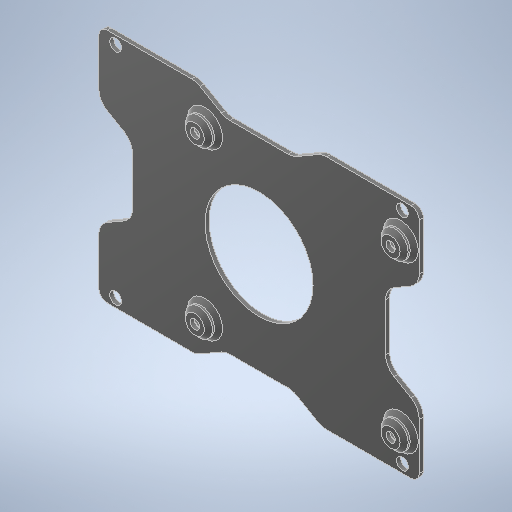
# Autodesk Inventor part: 3D_circuit-fix_raspberrypi
Saved by Autodesk Inventor 2025.1 (Build 291241020, 241B)
## iProperties
Created: 2024-07-24
Part Number: 3D_circuit-fix_raspberrypi
Material: 一般
Document SubType Name: Modeling
Designer: 8326d
Density: 1 g/cm^3
Appearance: 滑らか - 黒
Author: 8326d
## iProperties of the stored document 3D_circuit-fix_raspberrypi_3D プリント.ipt
Created: 2024-08-08
Part Number: 3D_circuit-fix_raspberrypi_3D プリント
Material: 一般
Document SubType Name: Modeling
Designer: 8326d
Density: 1 g/cm^3
Appearance: 既定
Author: 8326d
Autodesk Inventor part; units mm, degrees
ref_plane "YZ Plane" through (0, 0, 0) normal (1, 0, 0) x (0, 1, 0)
ref_plane "XZ Plane" through (0, 0, 0) normal (0, 1, 0) x (-1, 0, 0)
ref_plane "XY Plane" through (0, 0, 0) normal (0, 0, 1) x (1, 0, 0)
sketch "スケッチ1" plane through (0, 0, 0) normal (0, 0, 1) x (1, 0, 0)
  line L0 (-47.5, -35) -> (47.5, -35)
  line L1 (47.5, -35) -> (47.5, 35)
  line L2 (47.5, 35) -> (-47.5, 35)
  line L3 (-47.5, 35) -> (-47.5, -35)
  line L4 (-47.5, -35) -> (47.5, 35) construction
  line L5 (47.5, -35) -> (-47.5, 35) construction
  point P0 (0, 0)
  dimension "d0" = 95
  dimension "d1" = 70
  constraints: 12 end point, 2 midpoint, 2 parallel, 1 horizontal, 1 perpendicular
  measures "d0" distance of L2.end L1.end
  measures "d1" distance of L1.end L0.end
extrude "押し出し1" add sketch "スケッチ1" along normal blind 1.2
sketch "スケッチ2" plane through (0, 0, 1.2) normal (0, 0, 1) x (1, 0, 0)
  line L0 (-42.5, -32.5) -> (42.5, -32.5) construction
  line L1 (42.5, -32.5) -> (42.5, 32.5) construction
  line L2 (42.5, 32.5) -> (-42.5, 32.5) construction
  line L3 (-42.5, 32.5) -> (-42.5, -32.5) construction
  line L4 (-42.5, -32.5) -> (42.5, 32.5) construction
  line L5 (42.5, -32.5) -> (-42.5, 32.5) construction
  point P0 (0, 0)
  dimension "d4" = 85
  dimension "d5" = 65
  constraints: 12 end point, 2 midpoint, 2 parallel, 1 horizontal, 1 perpendicular
  measures "d4" distance of L2.end L1.end
  measures "d5" distance of L1.end L0.end
hole "穴1" at (-42.5, 32.5, 1.2) at (-42.5, -32.5, 1.2) at (42.5, -32.5, 1.2) at (42.5, 32.5, 1.2) direction (0, 0, -1) diameter 3.5 end through all
sketch "スケッチ3" plane through (0, 0, 1.2) normal (0, 0, 1) x (1, 0, 0)
  circle A0 centre (-16, -24.5) radius 4
  circle A1 centre (-16, 24.5) radius 4
  circle A2 centre (42, 24.5) radius 4
  circle A3 centre (42, -24.5) radius 4
  point P0 (0, 0)
  dimension "d13" = 8
  dimension "d14" = 8
  dimension "d15" = 8
  dimension "d16" = 8
  dimension "d17" = 49
  dimension "d21" = 58
  dimension "d22" = 24.5
  dimension "d52" = 16
  constraints: 4 centre point, 2 horizontal alignment, 2 vertical alignment
  measures "d13" diameter of A0
  measures "d14" diameter of A1
  measures "d15" diameter of A2
  measures "d16" diameter of A3
  measures "d17" distance of A0.centre A1.centre
  measures "d21" distance of A3.centre A0.centre
  measures "d22" vertical distance of A0.centre point (0, 0)
  measures "d52" horizontal distance of point (0, 0) A1.centre
extrude "押し出し2" add sketch "スケッチ3" along normal blind 3
chamfer "面取り1" distance 1.2 angle 45 8 edges at (-20, -24.5, 4.2) (-20, 24.5, 4.2) (38, 24.5, 4.2) (38, -24.5, 4.2) (-20, 24.5, 1.2) (-20, -24.5, 1.2) (38, 24.5, 1.2) (38, -24.5, 1.2)
sketch "スケッチ4" plane through (-16, -24.5, 4.2) normal (0, 0, 1) x (1, 0, 0)
  circle A0 centre (0, 49) radius 2.8 projected
  circle A1 centre (0, 0) radius 2.8 projected
  circle A2 centre (58, 0) radius 2.8 projected
  circle A3 centre (58, 49) radius 2.8 projected
  point P0 (16, 24.5)
hole "穴2" at (-16, 24.5, 4.2) at (-16, -24.5, 4.2) at (42, -24.5, 4.2) at (42, 24.5, 4.2) direction (0, 0, -1) diameter 2.8 end through all
sketch "スケッチ5" plane through (0, 0, 0) normal (0, 0, -1) x (-1, 0, 0)
  circle A0 centre (16, -24.5) radius 1.4 projected
  circle A1 centre (16, 24.5) radius 1.4 projected
  circle A2 centre (-42, 24.5) radius 1.4 projected
  circle A3 centre (-42, -24.5) radius 1.4 projected
  line L0 (16, -27.4445) -> (13.45, -25.9722)
  line L1 (13.45, -25.9722) -> (13.45, -23.0278)
  line L2 (13.45, -23.0278) -> (16, -21.5555)
  line L3 (16, -21.5555) -> (18.55, -23.0278)
  line L4 (18.55, -23.0278) -> (18.55, -25.9722)
  line L5 (18.55, -25.9722) -> (16, -27.4445)
  line L6 (16, 21.5555) -> (13.45, 23.0278)
  line L7 (13.45, 23.0278) -> (13.45, 25.9722)
  line L8 (13.45, 25.9722) -> (16, 27.4445)
  line L9 (16, 27.4445) -> (18.55, 25.9722)
  line L10 (18.55, 25.9722) -> (18.55, 23.0278)
  line L11 (18.55, 23.0278) -> (16, 21.5555)
  circle A4 centre (-42, -24.5) radius 2.8 projected
  line L12 (-42, -27.4445) -> (-44.55, -25.9722)
  line L13 (-44.55, -25.9722) -> (-44.55, -23.0278)
  line L14 (-44.55, -23.0278) -> (-42, -21.5555)
  line L15 (-42, -21.5555) -> (-39.45, -23.0278)
  line L16 (-39.45, -23.0278) -> (-39.45, -25.9722)
  line L17 (-39.45, -25.9722) -> (-42, -27.4445)
  line L18 (-42, 21.5555) -> (-44.55, 23.0278)
  line L19 (-44.55, 23.0278) -> (-44.55, 25.9722)
  line L20 (-44.55, 25.9722) -> (-42, 27.4445)
  line L21 (-42, 27.4445) -> (-39.45, 25.9722)
  line L22 (-39.45, 25.9722) -> (-39.45, 23.0278)
  line L23 (-39.45, 23.0278) -> (-42, 21.5555)
  point P0 (0, 0)
  dimension "d36" = 5.1
  dimension "d37" = 5.1
  dimension "d38" = 5.1
  dimension "d39" = 5.1
  constraints: 48 end point, 4 coincident, 4 vertical alignment, 52 other
  measures "d36" distance between parallel lines of L3 L0
  measures "d37" distance between parallel lines of L9 L6
  measures "d38" distance between parallel lines of L12 L15
  measures "d39" distance between parallel lines of L21 L18
extrude "押し出し3" cut sketch "スケッチ5" against normal blind 3 contours A2 | A3 | L0 L1 L2 L3 L4 L5 | L6 L7 L8 L9 L10 L11 | L16 A4 L17 L12 L13 L14 L15 | A4 L15 L16 | L16 L17 A4 | A4 L14 L15 | L17 L12 A4 | A4 L13 L14 | L12 L13 A4 | L18 L19 L20 L21 L22 L23
sketch "スケッチ6" plane through (0, 0, 3) normal (0, 0, -1) x (-1, 0, 0)
  line L0 (18.55, -23.0278) -> (18.55, -25.9722) projected
  line L1 (16, -21.5555) -> (18.55, -23.0278) projected
  line L2 (13.45, -23.0278) -> (16, -21.5555) projected
  line L3 (13.45, -25.9722) -> (13.45, -23.0278) projected
  line L4 (16, -27.4445) -> (13.45, -25.9722) projected
  line L5 (18.55, -25.9722) -> (16, -27.4445) projected
  circle A0 centre (16, -24.5) radius 1.4 projected
  line L6 (18.55, 25.9722) -> (18.55, 23.0278) projected
  line L7 (16, 27.4445) -> (18.55, 25.9722) projected
  line L8 (13.45, 25.9722) -> (16, 27.4445) projected
  line L9 (13.45, 23.0278) -> (13.45, 25.9722) projected
  line L10 (16, 21.5555) -> (13.45, 23.0278) projected
  line L11 (18.55, 23.0278) -> (16, 21.5555) projected
  circle A1 centre (16, 24.5) radius 1.4 projected
  circle A2 centre (-42, 24.5) radius 1.4 projected
  line L12 (-39.45, 25.9722) -> (-39.45, 23.0278) projected
  line L13 (-42, 27.4445) -> (-39.45, 25.9722) projected
  line L14 (-44.55, 25.9722) -> (-42, 27.4445) projected
  line L15 (-44.55, 23.0278) -> (-44.55, 25.9722) projected
  line L16 (-42, 21.5555) -> (-44.55, 23.0278) projected
  line L17 (-39.45, 23.0278) -> (-42, 21.5555) projected
  circle A3 centre (-42, -24.5) radius 1.4 projected
  line L18 (-44.55, -25.9722) -> (-44.55, -23.0278) projected
  line L19 (-42, -27.4445) -> (-44.55, -25.9722) projected
  line L20 (-39.45, -25.9722) -> (-42, -27.4445) projected
  line L21 (-39.45, -23.0278) -> (-39.45, -25.9722) projected
  line L22 (-42, -21.5555) -> (-39.45, -23.0278) projected
  line L23 (-44.55, -23.0278) -> (-42, -21.5555) projected
  line L24 (18.55, -23.0278) -> (18.55, -25.9722) projected
  line L25 (18.55, -24.6443) -> (14.85, -26.7805)
  line L26 (14.6, -26.6362) -> (14.6, -22.3638)
  line L27 (14.85, -22.2195) -> (18.55, -24.3557)
  line L28 (18.55, -25.9722) -> (16, -27.4445) projected
  line L29 (16, -21.5555) -> (18.55, -23.0278) projected
  circle A4 centre (16, -24.5) radius 1.4 projected
  line L30 (13.45, 25.9722) -> (16, 27.4445) projected
  line L31 (14.6, 26.6362) -> (14.6, 22.3638)
  line L32 (14.85, 22.2195) -> (18.55, 24.3557)
  line L33 (18.55, 25.9722) -> (18.55, 23.0278) projected
  line L34 (18.55, 24.6443) -> (14.85, 26.7805)
  line L35 (18.55, 23.0278) -> (16, 21.5555) projected
  line L36 (16, 27.4445) -> (18.55, 25.9722) projected
  circle A5 centre (16, 24.5) radius 1.4 projected
  line L37 (-43.4, 22.3638) -> (-43.4, 26.6362)
  line L38 (-43.15, 26.7805) -> (-39.45, 24.6443)
  line L39 (-39.45, 25.9722) -> (-39.45, 23.0278) projected
  line L40 (-39.45, 24.3557) -> (-43.15, 22.2195)
  line L41 (-42, 27.4445) -> (-39.45, 25.9722) projected
  line L42 (-39.45, 23.0278) -> (-42, 21.5555) projected
  circle A6 centre (-42, 24.5) radius 1.4 projected
  line L43 (-39.45, -24.6443) -> (-43.15, -26.7805)
  line L44 (-43.4, -26.6362) -> (-43.4, -22.3638)
  line L45 (-43.15, -22.2195) -> (-39.45, -24.3557)
  line L46 (-39.45, -25.9722) -> (-42, -27.4445) projected
  line L47 (-42, -21.5555) -> (-39.45, -23.0278) projected
  circle A7 centre (-42, -24.5) radius 1.4 projected
  point P0 (0, 0)
  point P1 (-39.45, 24.3557)
  point P2 (18.55, 24.3557)
  constraints: 24 end point, 24 point on line, 12 tangent, 8 parallel, 4 vertical
extrude "押し出し4" add sketch "スケッチ6" along normal blind 0.2 contours L0 L27 L2 L1 | L0 L5 L4 L25 | L26 L4 L3 L2 | L6 L34 L8 L7 | L6 L11 L10 L32 | L31 L10 L9 L8 | L38 L14 L13 L12 | L40 L12 L17 L16 | L37 L16 L15 L14 | L45 L23 L22 L21 | L43 L21 L20 L19 | L44 L19 L18 L23
fillet "フィレット1" radius 2.5 4 edges at (-47.5, -35, 0.6) (-47.5, 35, 0.6) (47.5, -35, 0.6) (47.5, 35, 0.6)
sketch "スケッチ7" plane through (0, 0, 1.2) normal (0, 0, 1) x (1, 0, 0)
  line L0 (45, 35) -> (-45, 35) projected
  line L1 (-10, 35) -> (10, 35)
  line L2 (10, 35) -> (10, 30)
  line L3 (10, 30) -> (-10, 30)
  line L4 (-10, 30) -> (-10, 35)
  line L5 (-10, 30) -> (-18.6603, 35)
  line L6 (10, 30) -> (18.6603, 35)
  line L7 (47.5, -32.5) -> (47.5, 32.5) projected
  line L8 (47.5, 10) -> (37.5, 10)
  line L9 (37.5, 10) -> (37.5, -10)
  line L10 (37.5, -10) -> (47.5, -10)
  line L11 (47.5, -10) -> (47.5, 10)
  line L12 (37.5, 10) -> (47.5, 15.7735)
  line L13 (47.5, -32.5) -> (47.5, 32.5) projected
  line L14 (47.5, 0) -> (37.5, 0)
  point P0 (0, 0)
  point P1 (0, 35)
  dimension "d45" = 20
  dimension "d46" = 5
  dimension "d47" = 30
  dimension "d48" = 30
  dimension "d53" = 20
  dimension "d54" = 10
  constraints: 24 end point, 5 midpoint, 5 parallel, 5 point on line, 2 horizontal, 2 perpendicular
  measures "d45" distance of L2.end L3.end
  measures "d46" distance of L1.end L2.end
  measures "d47" angle of L0 L6
  measures "d48" angle of L0 L5
  measures "d53" distance of L8.end L9.end
  measures "d54" distance of L8.start L8.end
extrude "押し出し5" cut sketch "スケッチ7" against normal through all contours L6 L2 L0 | L2 L3 L4 L0 | L4 L5 L0 | L14 L9 L8 L7 | L8 L12 L7
mirror "ミラー1" about plane through (0, 0, 0) normal (0, 1, 0) of "押し出し5"
mirror "ミラー2" about plane through (0, 0, 0) normal (1, 0, 0) of "押し出し5", "ミラー1"
fillet "フィレット2" radius 5 16 edges at (-18.6603, -35, 0.6) (-10, -30, 0.6) (10, -30, 0.6) (18.6603, -35, 0.6) (10, 30, 0.6) (-10, 30, 0.6) (-18.6603, 35, 0.6) (18.6603, 35, 0.6) (-47.5, -15.7735, 0.6) (-37.5, -10, 0.6) (-37.5, 10, 0.6) (-47.5, 15.7735, 0.6) (47.5, -15.7735, 0.6) (37.5, -10, 0.6) (37.5, 10, 0.6) (47.5, 15.7735, 0.6)
sketch "スケッチ8" plane through (0, 0, 1.2) normal (0, 0, 1) x (1, 0, 0)
  circle A0 centre (0, 0) radius 16
  dimension "d55" = 32
  constraints: 1 centre point, 1 coincident
  measures "d55" diameter of A0
extrude "押し出し6" cut sketch "スケッチ8" against normal through all
equation "\"d22\" = 0.5 * d17"
equation "\"d37\" = d36"
equation "\"d38\" = d36"
equation "\"d39\" = d36"
equation "\"d48\" = d47"
